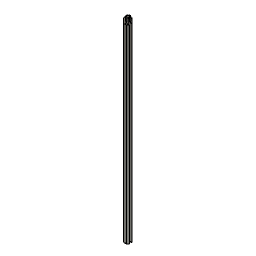
LEDC_baguettes_plexi_border2 v8 (Autodesk Fusion 360 design; units mm, degrees)
Autodesk Fusion 360 part; units mm, degrees
note: some values were not read from the file. Set by a fixed rule: which sketch regions a step uses.
sketch "Esquisse1" plane through (0, 0, 0) normal (0, 0, 1) x (1, 0, 0)
  line L0 (2, 12.2) -> (2, 7.2)
  line L1 (2, 7.2) -> (5.2, 7.2)
  line L2 (5.2, 7.2) -> (5.2, 12.2)
  line L3 (2, 12.2) -> (1.99, 12.2)
  line L4 (0, 0) -> (10.6066, 10.6066)
  line L5 (0, 0) -> (15, 0) construction
  line L6 (0, 10.21) -> (0, 6.2)
  line L7 (0, 6.2) -> (3.1, 3.1)
  line L8 (5.2, 12.2) -> (8.7, 8.7)
  line L9 (1.99, 12.2) -> (0, 10.21)
  point P0 (0, 12.2)
  dimension "d1" = 5
  dimension "d2" = 3.2
  dimension "d5" = 7.2
  dimension "d6" = 45
  dimension "d7" = 15
  dimension "d8" = 6
  dimension "d9" = 2
  dimension "d15" = 1.99
  dimension "d16" = 1.99
  constraint vertical L0
  constraint perpendicular L0 L1
  constraint perpendicular L1 L2
  constraint equal L0 L2
  constraint perpendicular L0 L3
  constraint horizontal L5
  constraint coincident L4.start L5.start
  constraint perpendicular L3 L6
  constraint coincident L4 L7.end
  constraint perpendicular L4 L7
  constraint coincident L4.start L6
  constraint coincident L4 L8.end
  constraint perpendicular L4 L8
  constraint coincident P0 L3
  constraint coincident P0 L6
  measures "d1" distance of L0.start L0.end
  measures "d2" distance of L0.end L1.end
  measures "d5" distance of L4.start L1
  measures "d6" angle of L4 L5
  measures "d7" distance of L4.start L4.end
  measures "d8" distance of P0 L6.end
  measures "d9" distance of L0.start P0
  measures "d15" distance of P0 L3.end
  measures "d16" distance of P0 L6.start
extrude "Extrusion1" add sketch "Esquisse1" along normal blind 254.5 makes body 1
mirror "Symétrie miroir1" about plane through (3.1, 3.1, 0) normal (-0.707107, 0.707107, 0) of bodies 1 merged
sketch "Esquisse4" plane through (0, 0, 254.5) normal (0, 0, 1) x (-1, 0, 0)
  line L0 (-2, -12.2) -> (-1.99, -12.2)
  line L1 (-1.99, -12.2) -> (0, -10.21)
  line L2 (0, -10.21) -> (0, -6.2)
  line L3 (0, -6.2) -> (-6.2, 0)
  line L4 (-6.2, 0) -> (-10.21, 0)
  line L5 (-10.21, 0) -> (-12.2, -1.99)
  line L6 (-12.2, -1.99) -> (-12.2, -2)
  line L7 (-12.2, -2) -> (-7.2, -2)
  line L8 (-7.2, -2) -> (-7.2, -5.2)
  line L9 (-7.2, -5.2) -> (-12.2, -5.2)
  line L10 (-12.2, -5.2) -> (-5.2, -12.2)
  line L11 (-5.2, -12.2) -> (-5.2, -7.2)
  line L12 (-5.2, -7.2) -> (-2, -7.2)
  line L13 (-2, -7.2) -> (-2, -12.2)
  line L14 (-5.2, -8.9) -> (-7.05, -8.9)
  line L15 (-7.05, -8.9) -> (-7.05, -7.05)
  line L16 (-7.05, -7.05) -> (-8.9, -7.05)
  line L17 (-8.9, -7.05) -> (-8.9, -5.2)
  line L18 (-5.2, -7.2) -> (-7.2, -5.2)
  line L19 (-3.5, -7.2) -> (-3.5, -5.35)
  line L20 (-3.5, -5.35) -> (-5.35, -5.35)
  line L21 (-5.35, -5.35) -> (-5.35, -3.5)
  line L22 (-5.35, -3.5) -> (-7.2, -3.5)
  point P0 (-7.2, -5.2)
  point P1 (-5.2, -7.2)
  point P2 (-7.2, -5.2)
  point P3 (-5.2, -7.2)
  dimension "d23" = 1.85
  constraint coincident L11 L14.start
  constraint perpendicular L11 L14
  constraint perpendicular L14 L15
  constraint perpendicular L11 L16
  constraint equal L15 L16
  constraint coincident L9 L17.end
  constraint equal L14 L17
  constraint coincident P3 P1
  constraint coincident P2 P0
  constraint symmetric P2 L18 P0
  constraint symmetric P3 L18 P1
  constraint symmetric L14.start L18 L19.start
  constraint symmetric L14.end L18 L19.end
  constraint symmetric L15.end L18 L20.end
  constraint symmetric L16.end L18 L21.end
  constraint symmetric L17.end L18 L22.end
  constraint coincident L16.end L17.start
  constraint perpendicular L16 L17
  constraint equal L14 L15
  measures "d23" distance of L14.start L14.end
extrude "Extrusion3" cut sketch "Esquisse4" against normal blind 4.5 contours L0 L1 L2 L3 L4 L5 L6 L7 L8 L12 L13 L19 L20 L21 L22 | L9 L10 L11 L14 L15 L16 L17 bodies 1
copy_body "Corps->Comp2" bodies 1 removing the originals makes body 2 in component "Component"
component "Component" placed x (1, 0, 0) y (0, 1, 0) z (0, 0, 1) at (0, 0, 0)
equation "d5 = d2 + 2 * d9"
equation "d8 = d1 + 1 mm"
equation "d16 = d15"
